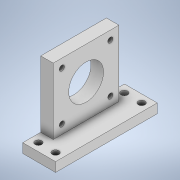
# Autodesk Inventor part: elbowmotorsupport
Saved by Autodesk Inventor 2022 (Build 260153000, 153)
## iProperties
Created: 2022-02-20
Part Number: elbowmotorsupport
Material: Genérico
Document SubType Name: Modeling
Designer: JK
Density: 1 g/cm^3
Appearance: Valor por defecto
Author: JK
Autodesk Inventor part; units mm, degrees
ref_plane "YZ Plane" through (0, 0, 0) normal (1, 0, 0) x (0, 1, 0)
ref_plane "XZ Plane" through (0, 0, 0) normal (0, 1, 0) x (-1, 0, 0)
ref_plane "XY Plane" through (0, 0, 0) normal (0, 0, 1) x (1, 0, 0)
sketch "Boceto1" plane through (0, 0, 0) normal (0, 1, 0) x (-1, 0, 0)
  line L0 (-10.5, 32.5) -> (10.5, 32.5)
  line L1 (10.5, 32.5) -> (10.5, -32.5)
  line L2 (10.5, -32.5) -> (-10.5, -32.5)
  line L3 (-10.5, -32.5) -> (-10.5, 32.5)
  line L4 (-10.5, 32.5) -> (10.5, -32.5) construction
  line L5 (10.5, 32.5) -> (-10.5, -32.5) construction
  circle A0 centre (5.5, 27.5) radius 2.15
  circle A1 centre (-5.5, 27.5) radius 2.15
  circle A2 centre (5.5, -27.5) radius 2.15
  circle A3 centre (-5.5, -27.5) radius 2.15
  point P0 (0, 0)
  dimension "d0" = 4.3
  dimension "d1" = 55
  dimension "d2" = 65
  dimension "d3" = 11
  dimension "d4" = 5
  dimension "d5" = 21
  dimension "d6" = 5
  constraints: 12 end point, 4 centre point, 3 equal radius, 2 horizontal alignment, 2 midpoint, 2 parallel, 2 vertical alignment, 1 horizontal, 1 perpendicular
  measures "d0" diameter of A0
  measures "d1" distance of A2.centre A0.centre
  measures "d2" distance of L0.end L1.end
  measures "d3" distance of A0.centre A1.centre
  measures "d4" distance from line of L1 A0.centre
  measures "d5" distance of L0.start L0.end
  measures "d6" distance from line of L0 A0.centre
extrude "Extrusión1" add sketch "Boceto1" along normal blind 6
sketch "Boceto2" plane through (0, 6, 0) normal (0, 1, 0) x (1, 0, 0)
  line L0 (-10.5, 32.5) -> (-10.5, -32.5) projected
  line L1 (-10.5, -21) -> (-2.5, -21)
  line L2 (-2.5, -21) -> (-2.5, 21)
  line L3 (-2.5, 21) -> (-10.5, 21)
  line L4 (-10.5, 21) -> (-10.5, -21)
  point P0 (0, 0)
  point P1 (-10.5, 21)
  dimension "d9" = 42
  dimension "d10" = 21
  dimension "d11" = 8
  constraints: 8 end point, 2 parallel, 1 horizontal, 1 perpendicular, 1 point on line
  measures "d9" distance between parallel lines of L3 L1
  measures "d10" distance from line of L1 point (0, 0)
  measures "d11" distance between parallel lines of L0 L2
extrude "Extrusión2" add sketch "Boceto2" along normal blind 42.3
sketch "Boceto3" plane through (-10.5, 0, -32.5) normal (-1, 0, 0) x (0, 0, 1)
  line L0 (11.5, 48.3) -> (53.5, 48.3) projected
  line L1 (53.5, 6) -> (53.5, 48.3) projected
  line L2 (11.5, 48.3) -> (53.5, 48.3)
  line L3 (53.5, 48.3) -> (53.5, 6.3)
  line L4 (53.5, 6.3) -> (11.5, 6.3)
  line L5 (11.5, 6.3) -> (11.5, 48.3)
  circle A0 centre (32.5, 27.3) radius 11.15
  point P0 (32.5, 0)
  dimension "d14" = 42
  dimension "d15" = 22.3
  dimension "d16" = 21
  dimension "d17" = 21
  constraints: 8 end point, 2 parallel, 1 centre point, 1 horizontal, 1 perpendicular, 1 point on line
  measures "d14" distance of L4.end L0.start
  measures "d15" diameter of A0
  measures "d16" distance from line of L5 A0.centre
  measures "d17" distance from line of A0.centre L4
extrude "Extrusión3" cut sketch "Boceto3" against normal through all contours A0
sketch "Boceto4" plane through (-10.5, 0, -32.5) normal (-1, 0, 0) x (0, 0, 1)
  circle A0 centre (17, 42.8) radius 1.65
  circle A1 centre (32.5, 27.3) radius 11.15 projected
  point P0 (32.5, 0)
  dimension "d20" = 15.5
  dimension "d22" = 15.5
  dimension "d23" = 3.3
  constraints: 1 centre point
  measures "d20" horizontal distance of A0.centre A1.centre
  measures "d22" horizontal distance of A1.centre A0.centre
  measures "d23" diameter of A0
extrude "Extrusión4" cut sketch "Boceto4" against normal through all contours A0
chamfer "Chaflán1" distance 1.5 angle 45 1 edges at (-10.5, 42.8, -17.15)
pattern_circular "Patrón circular1" count 4 over 360 about axis through (-10.5, 27.3, 0) along (1, 0, 0) of "Extrusión4", "Chaflán1"
